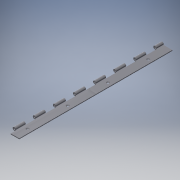
# Autodesk Inventor part: SIDE 2
Saved by Autodesk Inventor 2016 (Build 200138000, 138)
## iProperties
Created: 2015-09-17
Part Number: SIDE 2
Material: Steel, Mild
Document SubType Name: Modeling
Designer: testing
Density: 7.85 g/cm^3
Appearance: Metal-Steel
Mass: 86.9641 g
Surface Area: 161.988 cm^2
Volume: 11.0782 cm^3
User Status: have
Author: testing
Autodesk Inventor part; units mm, degrees
ref_plane "YZ Plane" through (0, 0, 0) normal (1, 0, 0) x (0, 1, 0)
ref_plane "XZ Plane" through (0, 0, 0) normal (0, 1, 0) x (-1, 0, 0)
ref_plane "XY Plane" through (0, 0, 0) normal (0, 0, 1) x (1, 0, 0)
sketch "Sketch2" plane through (0, 0, 0) normal (0, 1, 0) x (-1, 0, 0)
  arc A0 (0, -1.5) -> (-1.3365, -0.681) centre (0, 0) ccw
  arc A1 (0, -3) -> (-2.673, -1.362) centre (0, 0) ccw
  line L0 (0, -3) -> (-20, -3)
  line L1 (-20, -3) -> (-20, -1.5)
  line L2 (-20, -1.5) -> (0, -1.5)
  line L3 (-1.3365, -0.681) -> (-2.673, -1.362)
  dimension "d0" = 1.5
  dimension "d1" = 1.5
  dimension "d2" = 20
  dimension "d3" = 3
  dimension "d4" = 27
  constraints: 8 end point, 4 point on circle, 3 coincident, 2 centre point, 1 horizontal, 1 parallel, 1 perpendicular, 1 point on line, 1 tangent
  measures "d0" distance of L0.end L1.end
  measures "d1" radial gap between concentric circles of A1 A0
  measures "d2" distance from line of point (0, 0) L1
  measures "d3" diameter of A0
  measures "d4" angle of L2 L3
extrude "Extrusion1" add sketch "Sketch2" along normal blind 304.8
sketch "Sketch3" plane through (20, 0, -3) normal (0, 0, -1) x (-1, 0, 0)
  line L0 (0, 0) -> (20, 0) projected
  line L1 (23, 50) -> (17, 50)
  line L2 (17, 50) -> (17, 30)
  line L3 (17, 30) -> (23, 30)
  line L4 (23, 30) -> (23, 50)
  line L5 (17, 0) -> (17, 304.8) projected
  dimension "d8" = 20
  dimension "d9" = 6
  dimension "d24" = 30
  constraints: 8 end point, 2 parallel, 1 horizontal, 1 perpendicular, 1 point on line
  measures "d8" distance of L3.end L1.start
  measures "d9" distance of L2.end L3.end
  measures "d24" distance between parallel lines of L0 L3
extrude "Extrusion2" cut sketch "Sketch3" against normal through all
pattern_linear "Rectangular Pattern1" count 25 spacing 40 along (0, 1, 0) of "Extrusion2"
sketch "Sketch5" plane through (20, 0, -3) normal (0, 0, -1) x (-1, 0, 0)
  line L0 (0, 0) -> (20, 0) projected
  line L1 (17, 0) -> (23, 0)
  line L2 (23, 0) -> (23, 10)
  line L3 (23, 10) -> (17, 10)
  line L4 (17, 10) -> (17, 0)
  point P0 (17, 30)
  dimension "d25" = 10
  dimension "d26" = 6
  constraints: 8 end point, 2 parallel, 1 horizontal, 1 horizontal alignment, 1 perpendicular, 1 vertical alignment
  measures "d25" distance between parallel lines of L3 L0
  measures "d26" distance of L2.end L3.end
extrude "Extrusion3" cut sketch "Sketch5" against normal through all
sketch "Sketch4" plane through (20, 0, -1.5) normal (0, 0, 1) x (1, 0, 0)
  line L0 (0, 0) -> (0, 304.8) projected
  line L1 (0, 304.8) -> (-20, 304.8) projected
  point P0 (-8, -615.2)
  point P1 (-8, -535.2)
  point P2 (-8, -455.2)
  point P3 (-8, -375.2)
  point P4 (-8, -295.2)
  point P5 (-8, -215.2)
  point P6 (-8, -135.2)
  point P7 (-8, -55.2)
  point P8 (-8, 24.8)
  point P9 (-8, 104.8)
  point P10 (-8, 184.8)
  point P11 (-8, 264.8)
  point P12 (-17, 1000)
  point P13 (-20, 304.8)
  dimension "d15" = 8
  dimension "d29" = 40
  dimension "d30" = 80
  dimension "d31" = 80
  dimension "d32" = 80
  dimension "d33" = 80
  dimension "d34" = 80
  dimension "d35" = 80
  dimension "d36" = 80
  dimension "d37" = 80
  dimension "d38" = 80
  dimension "d39" = 80
  dimension "d40" = 80
  constraints: 11 vertical alignment, 1 other
  measures "d15" distance from line of L0 point (-8, -615.2)
  measures "d30" distance of point (-8, 184.8) point (-8, 264.8)
  measures "d31" distance of point (-8, 104.8) point (-8, 184.8)
  measures "d32" distance of point (-8, 24.8) point (-8, 104.8)
  measures "d33" distance of point (-8, -55.2) point (-8, 24.8)
  measures "d34" distance of point (-8, -135.2) point (-8, -55.2)
  measures "d35" distance of point (-8, -215.2) point (-8, -135.2)
  measures "d36" distance of point (-8, -295.2) point (-8, -215.2)
  measures "d37" distance of point (-8, -375.2) point (-8, -295.2)
  measures "d38" distance of point (-8, -455.2) point (-8, -375.2)
  measures "d39" distance of point (-8, -535.2) point (-8, -455.2)
  measures "d40" distance of point (-8, -615.2) point (-8, -535.2)
hole "Hole1" at (12, -615.2, -1.5) at (12, -535.2, -1.5) at (12, -455.2, -1.5) at (12, -375.2, -1.5) at (12, -295.2, -1.5) at (12, -215.2, -1.5) at (12, -135.2, -1.5) at (12, -55.2, -1.5) at (12, 24.8, -1.5) at (12, 104.8, -1.5) at (12, 184.8, -1.5) at (12, 264.8, -1.5) direction (0, 0, -1) diameter 3 end through all countersink diameter 6 countersink angle 90
equation "\"d1\" = d0"
equation "\"d31\" = d30"
equation "\"d32\" = d30"
equation "\"d33\" = d30"
equation "\"d34\" = d30"
equation "\"d35\" = d30"
equation "\"d36\" = d30"
equation "\"d37\" = d36"
equation "\"d38\" = d37"
equation "\"d39\" = d38"
equation "\"d40\" = d39"
body "Solid1"
